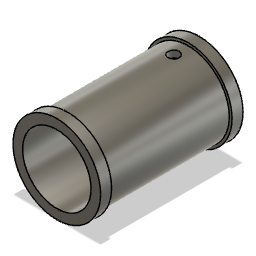
GasChargingCryoarmGuideForCartridge v4 (Autodesk Fusion 360 design; units mm, degrees)
Autodesk Fusion 360 part; units mm, degrees
sketch "Skizze3" plane through (0, 0, 0) normal (0, 1, 0) x (1, 0, 0)
  line L0 (0, 0) -> (0, 13)
  line L1 (0, 13) -> (8, 13)
  line L2 (8, 13) -> (8, 11)
  line L3 (8, 11) -> (7.5, 11)
  line L4 (7.5, 11) -> (7.5, 0)
  line L5 (1.75, 0) -> (22.5, 0)
  line L6 (0, 0) -> (0, -13)
  line L7 (0, -13) -> (8, -13)
  line L8 (8, -11) -> (7.5, -11)
  line L9 (7.5, -11) -> (7.5, 0)
  line L10 (8, -13) -> (8, -11)
  dimension "d14" = 13
  dimension "d15" = 8
  dimension "d16" = 2
  dimension "d17" = 0.5
  constraint coincident L0.start L6.start
  constraint vertical L0
  constraint perpendicular L0 L1
  constraint perpendicular L1 L2
  constraint perpendicular L2 L3
  constraint perpendicular L1 L4
  constraint symmetric L0.start L5 L6.start
  constraint symmetric L0.end L5 L6.end
  constraint symmetric L1.end L5 L7.end
  constraint symmetric L2.end L5 L8.start
  constraint symmetric L3.end L5 L8.end
  constraint symmetric L4.end L5 L9.end
  measures "d14" distance of L0.start L0.end
  measures "d15" distance of L0.end L1.end
  measures "d16" distance of L1.end L2.end
  measures "d17" distance of L2.end L3.end
revolve "Drehen1" add sketch "Skizze3" angle 360 about axis through (0, 0, 0) along (0, 0, 1)
hole "Bohrung1" at (0, 0, 13) direction (0, 0, -1) diameter 12.5 end through all
ref_plane "Arbeitsebene1" through (0, 7.5, 0) normal (0, 1, 0) x (0, 0, 1)
sketch "Skizze5" plane through (0, 7.5, 0) normal (0, 1, 0) x (1, 0, 0)
  circle A0 centre (0, 8.3) radius 1
  dimension "d24" = 2
  measures "d24" diameter of A0
extrude "Extrusion3" cut sketch "Skizze5" against normal blind 3
component "Component" placed x (1, 0, 0) y (0, 1, 0) z (0, 0, 1) at (0, 0, 0)
